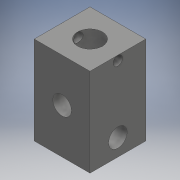
# Autodesk Inventor part: Centerhoved
Saved by Autodesk Inventor 2018 (Build 220112000, 112)
## iProperties
Created: 2018-01-29
Part Number: Centerhoved
Material: PC/ABS Plastic
Document SubType Name: Modeling
Designer: MikkelS
Density: 0.357273 g/cm^3
Appearance: Smooth - White
Author: MikkelS
Autodesk Inventor part; units mm, degrees
ref_plane "YZ Plane" through (0, 0, 0) normal (1, 0, 0) x (0, 1, 0)
ref_plane "XZ Plane" through (0, 0, 0) normal (0, 1, 0) x (-1, 0, 0)
ref_plane "XY Plane" through (0, 0, 0) normal (0, 0, 1) x (1, 0, 0)
sketch "Sketch1" plane through (0, 0, 0) normal (0, 0, 1) x (1, 0, 0)
  line L0 (0, 0) -> (0, 36)
  line L1 (0, 36) -> (36, 36)
  line L2 (36, 36) -> (36, 0)
  line L3 (36, 0) -> (0, 0)
  dimension "d0" = 36
  dimension "d1" = 36
  constraints: 8 end point, 3 perpendicular, 1 vertical
  measures "d0" distance of L0.start L0.end
  measures "d1" distance of L0.end L1.end
extrude "Extrusion1" add sketch "Sketch1" along normal blind 57
sketch "Sketch2" plane through (0, 0, 57) normal (0, 0, 1) x (1, 0, 0)
  circle A0 centre (18, 18) radius 8
  dimension "d4" = 16
  constraints: 1 centre point
  measures "d4" diameter of A0
hole "Hole1" at (18, 18, 57) direction (0, 0, -1) diameter 16 depth 17
sketch "Sketch3" plane through (36, 0, 0) normal (1, 0, 0) x (0, 0, -1)
  circle A0 centre (-11, 18) radius 6
  dimension "d43" = 12
  constraints: 1 centre point
  measures "d43" diameter of A0
hole "Hole2" at (36, 18, 11) direction (-1, 0, 0) diameter 12 end through all
sketch "Sketch4" plane through (0, 36, 0) normal (0, 1, 0) x (1, 0, 0)
  circle A0 centre (18, -29) radius 6
  dimension "d46" = 12
  constraints: 1 centre point
  measures "d46" diameter of A0
hole "Hole3" at (18, 36, 29) direction (0, -1, 0) diameter 12 end through all
sketch "Sketch5" plane through (36, 0, 0) normal (1, 0, 0) x (0, 0, -1)
  circle A0 centre (-53.9561, 18) radius 3
  point P0 (0, 0)
  dimension "d41" = 6
  constraints: 1 centre point
  measures "d41" diameter of A0
hole "Hole4" at (36, 18, 53.9561) direction (-1, 0, 0) diameter 6 end through all
body "Solid1"
